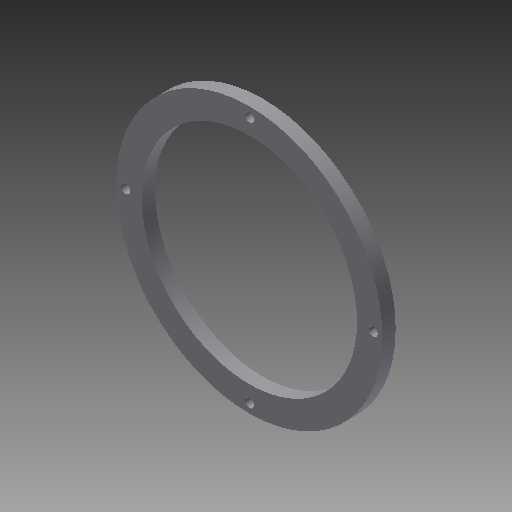
# Autodesk Inventor part: rotBase
Saved by Autodesk Inventor 2017 (Build 210142000, 142)
## iProperties
Created: 2016-09-29
Part Number: rotBase
Material: Generic
Document SubType Name: Modeling
Designer: Bardo91
Density: 1 g/cm^3
Appearance: Default
Author: Bardo91
Autodesk Inventor part; units mm, degrees
ref_plane "YZ Plane" through (0, 0, 0) normal (1, 0, 0) x (0, 1, 0)
ref_plane "XZ Plane" through (0, 0, 0) normal (0, 1, 0) x (-1, 0, 0)
ref_plane "XY Plane" through (0, 0, 0) normal (0, 0, 1) x (1, 0, 0)
sketch "Sketch1" plane through (0, 0, 0) normal (0, 0, 1) x (1, 0, 0)
  circle A0 centre (0, 0) radius 40.5
  circle A1 centre (0, 0) radius 43
  circle A2 centre (0, 0) radius 50
  line L0 (0, 50) -> (0, 43)
  circle A3 centre (0, 46.5) radius 1.75
  circle A4 centre (-46.5, 0) radius 1.75
  circle A5 centre (0, -46.5) radius 1.75
  circle A6 centre (46.5, 0) radius 1.75
  dimension "d1" = 86
  dimension "d2" = 100
  dimension "d0" = 81
  dimension "d3" = 3.5
  dimension "d6" = 360
  constraints: 5 centre point, 3 coincident, 2 end point, 2 vertical alignment, 1 midpoint, 1 vertical, 13 other
  measures "d0" diameter of A0
  measures "d3" diameter of A3
extrude "Extrusion1" add sketch "Sketch1" along normal blind 5 contours A1 | A2
body "Solid1"
